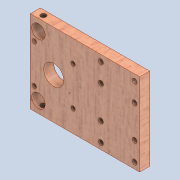
# Autodesk Inventor part: 0005-10-027 suport nema Z
Saved by Autodesk Inventor 2020 (Build 240168000, 168)
## iProperties
Created: 2020-12-18
Part Number: 0005-10-027 suport nema Z
Material: Wood (Maple)
Document SubType Name: Modeling
Designer: Iulian Bors
Density: 0.67 g/cm^3
Appearance: White Oak - Natural Medium Gloss
Mass: 28.2154 g
Surface Area: 151.277 cm^2
Volume: 42.1125 cm^3
Author: Iulian Bors
Subject: 027
Autodesk Inventor part; units mm, degrees
ref_plane "YZ Plane" through (0, 0, 0) normal (1, 0, 0) x (0, 1, 0)
ref_plane "XZ Plane" through (0, 0, 0) normal (0, 1, 0) x (-1, 0, 0)
ref_plane "XY Plane" through (0, 0, 0) normal (0, 0, 1) x (1, 0, 0)
sketch "Sketch1" plane through (0, 0, 0) normal (0, 0, 1) x (1, 0, 0)
  line L0 (-43.75, 33) -> (43.75, 33)
  line L1 (43.75, 33) -> (43.75, -33)
  line L2 (43.75, -33) -> (-43.75, -33)
  line L3 (-43.75, -33) -> (-43.75, 33)
  point P0 (0, 0)
  point P1 (0, 33)
  point P2 (-43.75, 0)
  dimension "d0" = 87.5
  dimension "d1" = 66
  constraints: 8 end point, 2 midpoint, 2 parallel, 1 horizontal, 1 horizontal alignment, 1 perpendicular, 1 vertical alignment
  measures "d0" distance of L0.start L0.end
  measures "d1" distance of L2.end L0.start
extrude "Extrusion1" add sketch "Sketch1" along normal blind 8
sketch "Sketch4" plane through (0, 0, 8) normal (0, 0, 1) x (1, 0, 0)
  line L0 (43.75, 33) -> (-43.75, 33) projected
  line L1 (-43.75, 33) -> (-43.75, -33) projected
  circle A0 centre (-37.25, 24) radius 5.4
  circle A1 centre (-37.25, -24) radius 5.4
  line L2 (-43.75, -33) -> (43.75, -33) projected
  point P0 (0, 0)
  dimension "d27" = 6.5
  dimension "d28" = 9
  dimension "d29" = 10.8
  dimension "d30" = 9
  constraints: 2 centre point, 1 equal radius, 1 vertical alignment
  measures "d27" distance from line of A0.centre L1
  measures "d28" distance from line of L0 A0.centre
  measures "d29" diameter of A0
  measures "d30" distance from line of L2 A1.centre
extrude "Extrusion4" cut sketch "Sketch4" against normal through all
sketch "Sketch5" plane through (0, 0, 8) normal (0, 0, 1) x (1, 0, 0)
  circle A0 centre (-25.0012, 0) radius 4
  circle A1 centre (-25.0012, 0) radius 8
  line L0 (-43.75, 33) -> (-43.75, -33) projected
  line L1 (43.75, 33) -> (-43.75, 33) projected
  circle A2 centre (-25.0012, 0) radius 4 projected
  circle A3 centre (-25.0012, 0) radius 7 projected
  point P0 (0, 0)
  point P1 (-43.75, 0)
  dimension "d24" = 16
  dimension "d33" = 18.7488
  constraints: 2 centre point, 2 horizontal alignment, 1 concentric, 1 midpoint
  measures "d24" diameter of A1
  measures "d33" distance from line of A0.centre L0
extrude "Extrusion5" cut sketch "Sketch5" against normal through all contours A0 | A1 | A3
sketch "Sketch6" plane through (0, 0, 8) normal (0, 0, 1) x (1, 0, 0)
  circle A0 centre (-40.5012, 15.5) radius 1.75
  circle A1 centre (-9.5012, 15.5) radius 1.75
  circle A2 centre (-9.5012, -15.5) radius 1.75
  circle A3 centre (-40.5012, -15.5) radius 1.75
  line L0 (-40.5012, 15.5) -> (-9.5012, 15.5)
  line L1 (-9.5012, 15.5) -> (-9.5012, -15.5)
  line L2 (-9.5012, -15.5) -> (-40.5012, -15.5)
  line L3 (-40.5012, -15.5) -> (-40.5012, 15.5)
  line L4 (-40.5012, 15.5) -> (-9.5012, -15.5) construction
  line L5 (-9.5012, 15.5) -> (-40.5012, -15.5) construction
  circle A4 centre (-25.0012, 0) radius 8 projected
  line L6 (-43.75, 33) -> (-43.75, -33) projected
  line L7 (43.75, 33) -> (-43.75, 33) projected
  circle A5 centre (-40.5012, -15.5) radius 2.75 projected
  circle A6 centre (-9.5012, 15.5) radius 3 projected
  point P0 (0, 0)
  point P1 (-25.0012, 0)
  dimension "d35" = 3.5
  dimension "d36" = 31
  constraints: 12 end point, 4 centre point, 4 coincident, 3 equal radius, 3 midpoint, 3 parallel, 1 horizontal, 1 perpendicular
  measures "d35" diameter of A1
  measures "d36" distance of L0.start L0.end
extrude "Extrusion6" cut sketch "Sketch6" against normal through all contours L0 L3 A0 | A0 L3 L0 | L0 L1 A1 | A1 L1 L0 | L3 L2 A3 | A3 L2 L3 | L1 L2 A2 | A2 L2 L1
sketch "Sketch8" plane through (0, 0, 0) normal (0, 0, -1) x (-1, 0, 0)
  line L0 (-43.75, 33) -> (43.75, 33) projected
  line L1 (-43.75, -33) -> (-43.75, 33) projected
  point P0 (0, 0)
  point P1 (-39.75, 28)
  point P2 (-39.75, 13)
  point P3 (-39.75, -13)
  point P4 (-39.75, -28)
  dimension "d38" = 5
  dimension "d39" = 15
  dimension "d40" = 26
  dimension "d41" = 15
  dimension "d42" = 4
  constraints: 3 vertical alignment
  measures "d38" distance from line of L0 point (-39.75, 28)
  measures "d39" distance of point (-39.75, 13) point (-39.75, 28)
  measures "d40" distance of point (-39.75, -13) point (-39.75, 13)
  measures "d41" distance of point (-39.75, -28) point (-39.75, -13)
  measures "d42" distance from line of L1 point (-39.75, 28)
hole "Hole1" at (39.75, 28, 0) direction (0, 0, 1) diameter 4 end through all
pattern_linear "Rectangular Pattern1" count 2 spacing 15 along (0, -1, 0) count 2 spacing 41 along (0, -1, 0) of "Hole1"
pattern_linear "Rectangular Pattern2" count 2 spacing 27 along (-1, 0, 0) of "Hole1", "Rectangular Pattern1"
sketch "Sketch9" plane through (-43.75, -33, 0) normal (0, -1, 0) x (1, 0, 0)
  line L0 (0, 0) -> (0, 8) projected
  point P0 (43.75, 0)
  point P1 (6.5, 4)
  point P2 (0, 4)
  dimension "d59" = 6.5
  constraints: 1 horizontal alignment, 1 midpoint
  measures "d59" horizontal distance of L0.end point (6.5, 4)
hole "Hole2" at (-37.25, -33, 4) direction (0, 1, 0) diameter 4.134 depth 7.45 tip angle 118 thread size "M5x0.8" class "6H" standard "ISO Metric profile"
sketch "Sketch10" plane through (-43.75, 33, 0) normal (0, 1, 0) x (1, 0, 0)
  circle A0 centre (6.5, -4) radius 2.067 projected
  point P0 (43.75, 0)
  constraints: 1 coincident
hole "Hole3" at (-37.25, 33, 4) direction (0, -1, 0) diameter 4.134 depth 7.45 tip angle 118 thread size "M5x0.8" class "6H" standard "ISO Metric profile"
equation "\"d30\" = d28"
body "Solid1"
